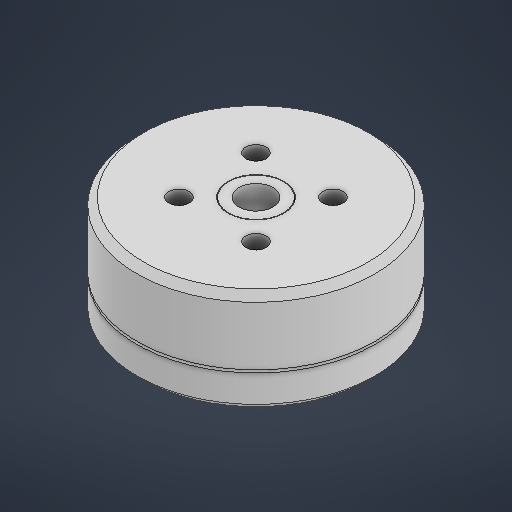
# Autodesk Inventor part: Motor
Saved by Autodesk Inventor 2026.1 (Build 301233020, 233B)
## iProperties
Created: 2026-05-23
Part Number: Motor
Material: Generic
Document SubType Name: Modeling
Designer: InventorKid
Density: 1 g/cm^3
Appearance: Default
Author: InventorKid
Autodesk Inventor part; units mm, degrees
ref_plane "YZ Plane" through (0, 0, 0) normal (1, 0, 0) x (0, 1, 0)
ref_plane "XZ Plane" through (0, 0, 0) normal (0, 1, 0) x (-1, 0, 0)
ref_plane "XY Plane" through (0, 0, 0) normal (0, 0, 1) x (1, 0, 0)
sketch "Sketch1" plane through (0, 0, 0) normal (0, 1, 0) x (-1, 0, 0)
  circle A0 centre (0, 0) radius 17.5
  circle A1 centre (0, 0) radius 2.5
  circle A2 centre (9.5, 0) radius 1.5
  circle A3 centre (0, -8) radius 1.5
  circle A4 centre (-9.5, 0) radius 1.5
  circle A5 centre (0, 8) radius 1.5
  dimension "d0" = 35
  dimension "d1" = 5
  dimension "d2" = 3
  dimension "d3" = 16
  dimension "d4" = 8
  dimension "d5" = 19
  dimension "d6" = 9.5
  constraints: 6 centre point, 3 equal radius, 2 coincident, 2 horizontal alignment, 2 vertical alignment
  measures "d0" diameter of A0
  measures "d1" diameter of A1
  measures "d2" diameter of A2
  measures "d3" distance of A3.centre A5.centre
  measures "d4" distance of point (0, 0) A5.centre
  measures "d5" distance of A4.centre A2.centre
  measures "d6" distance of point (0, 0) A4.centre
extrude "Extrusion1" add sketch "Sketch1" along normal blind 5
sketch "Sketch2" plane through (0, 5, 0) normal (0, 1, 0) x (1, 0, 0)
  circle A0 centre (0, 0) radius 4
  circle A1 centre (0, 0) radius 2.5
  dimension "d9" = 8
  dimension "d10" = 5
  constraints: 2 centre point, 2 coincident
  measures "d9" diameter of A0
  measures "d10" diameter of A1
extrude "Extrusion2" add sketch "Sketch2" along normal blind 10
chamfer "Chamfer1" distance 1 angle 45 1 edges at (17.5, 0, 0)
sketch "Sketch3" plane through (0, 15, 0) normal (0, 1, 0) x (1, 0, 0)
  circle A0 centre (0, 0) radius 17.5
  circle A1 centre (0, 0) radius 4.1
  circle A2 centre (0, 0) radius 2.5 construction
  circle A3 centre (0, 0) radius 8 construction
  circle A4 centre (-5.6569, -5.6569) radius 1.5
  circle A5 centre (-5.6569, 5.6569) radius 1.5
  circle A6 centre (5.6569, 5.6569) radius 1.5
  circle A7 centre (5.6569, -5.6569) radius 1.5
  dimension "d16" = 35
  dimension "d17" = 8.2
  dimension "d18" = 16
  dimension "d19" = 3
  dimension "d20" = 90
  constraints: 7 centre point, 3 coincident, 3 equal radius, 3 point on circle, 2 horizontal alignment, 2 vertical alignment
  measures "d16" diameter of A0
  measures "d17" diameter of A1
  measures "d18" diameter of A3
  measures "d19" diameter of A4
extrude "Extrusion3" add sketch "Sketch3" against normal blind 9.6
chamfer "Chamfer2" distance 1 angle 45 1 edges at (-17.5, 15, 0)
sketch "Sketch4" plane through (0, 0, 0) normal (0, -1, 0) x (1, 0, 0)
  line L0 (-10.4797, -6.9441) -> (-6.9441, -10.4797)
  line L1 (-10.4797, -6.9441) -> (-5.4797, -6.9441) construction
  line L2 (-6.9441, -10.4797) -> (-14.0152, -17.5507)
  line L3 (-14.0152, -17.5507) -> (-17.5507, -14.0152)
  line L4 (-17.5507, -14.0152) -> (-10.4797, -6.9441)
  line L5 (-15.783, -15.783) -> (0, 0) construction
  circle A0 centre (0, 0) radius 17.5 projected
  point P0 (-14.0152, -10.4797)
  dimension "d26" = 45
  dimension "d27" = 5
  dimension "d28" = 10
  constraints: 12 end point, 4 perpendicular, 2 midpoint, 1 equal length, 1 horizontal, 2 other
  measures "d26" angle of L0 L1
  measures "d27" distance between parallel lines of L2 L4
  measures "d28" distance between parallel lines of L0 L3
extrude "Extrusion4" add sketch "Sketch4" against normal blind 4 contours L0 L2 A0 L4 | A0 L2 L3 L4 picked at (-10.125, -9.731)
fillet "Fillet1" radius 1 4 edges at (-15.4255, 0, -11.89) (-15.783, 4, -12.2474) (-11.89, 0, -15.4255) (-12.2474, 4, -15.783)
body "Solid1"
